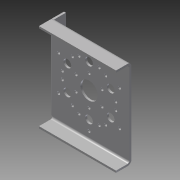
# Autodesk Inventor part: Plate 2 (Back)
Saved by Autodesk Inventor 2014 (Build 180170000, 170)
## iProperties
Created: 2014-01-12
Part Number: Plate 2 (Back)
Material: Steel
Document SubType Name: Sheet Metal
Designer: Andrew Toennies
Density: 7.85 g/cm^3
Sheet Metal Rule: Default
Appearance: Steel
Mass: 879.453 g
Surface Area: 760.069 cm^2
Volume: 112.032 cm^3
Author: Andrew Toennies
Autodesk Inventor part; units mm, degrees
ref_plane "YZ Plane" through (0, 0, 0) normal (1, 0, 0) x (0, 1, 0)
ref_plane "XZ Plane" through (0, 0, 0) normal (0, 1, 0) x (-1, 0, 0)
ref_plane "XY Plane" through (0, 0, 0) normal (0, 0, 1) x (1, 0, 0)
sketch "Sketch1" plane through (0, 0, 0) normal (0, 0, 1) x (1, 0, 0)
  circle A0 centre (0, 0) radius 66.675 construction
  circle A1 centre (0, 0) radius 14.2875
  circle A2 centre (0, 41.275) radius 6.3881
  line L0 (0, 0) -> (0, 41.275) construction
  circle A3 centre (0, 41.275) radius 16.637 construction
  circle A4 centre (0, 57.912) radius 2.3812
  circle A5 centre (16.637, 41.275) radius 2.3812
  circle A6 centre (0, 24.638) radius 2.3812
  circle A7 centre (-16.637, 41.275) radius 2.3813
  line L1 (0, 41.275) -> (0, 57.912) construction
  line L2 (-16.637, 41.275) -> (16.637, 41.275) construction
  circle A8 centre (-50.1533, 28.956) radius 2.3812
  circle A9 centre (-44.0637, 6.2294) radius 2.3813
  circle A10 centre (-35.7452, 20.6375) radius 6.3881
  circle A11 centre (-27.4267, 35.0456) radius 2.3812
  circle A12 centre (-21.3371, 12.319) radius 2.3812
  circle A13 centre (-50.1533, -28.956) radius 2.3812
  circle A14 centre (-27.4267, -35.0456) radius 2.3813
  circle A15 centre (-35.7452, -20.6375) radius 6.3881
  circle A16 centre (-44.0637, -6.2294) radius 2.3812
  circle A17 centre (-21.3371, -12.319) radius 2.3812
  circle A18 centre (0, -57.912) radius 2.3812
  circle A19 centre (16.637, -41.275) radius 2.3813
  circle A20 centre (0, -41.275) radius 6.3881
  circle A21 centre (-16.637, -41.275) radius 2.3812
  circle A22 centre (0, -24.638) radius 2.3812
  circle A23 centre (50.1533, -28.956) radius 2.3812
  circle A24 centre (44.0637, -6.2294) radius 2.3813
  circle A25 centre (35.7452, -20.6375) radius 6.3881
  circle A26 centre (27.4267, -35.0456) radius 2.3812
  circle A27 centre (21.3371, -12.319) radius 2.3812
  circle A28 centre (50.1533, 28.956) radius 2.3812
  circle A29 centre (27.4267, 35.0456) radius 2.3813
  circle A30 centre (35.7452, 20.6375) radius 6.3881
  circle A31 centre (44.0637, 6.2294) radius 2.3812
  circle A32 centre (21.3371, 12.319) radius 2.3812
  line L3 (-66.675, 66.675) -> (66.675, 66.675)
  line L4 (66.675, 66.675) -> (66.675, -66.675)
  line L5 (66.675, -66.675) -> (-66.675, -66.675)
  line L6 (-66.675, -66.675) -> (-66.675, 66.675)
  dimension "d2" = 133.35
  dimension "d3" = 28.575
  dimension "d4" = 12.7762
  dimension "d5" = 41.275
  dimension "d6" = 33.274
  dimension "d7" = 4.7625
  dimension "d8" = 4.7625
  dimension "d9" = 4.7625
  dimension "d10" = 4.7625
  dimension "d11" = 360
  measures "d2" diameter of A0
  measures "d3" diameter of A1
  measures "d4" diameter of A2
  measures "d5" distance of L0.start L0.end
  measures "d6" diameter of A3
  measures "d7" diameter of A4
  measures "d8" diameter of A5
  measures "d9" diameter of A6
  measures "d10" diameter of A7
extrude "Plate1" add sketch "Sketch1" along normal blind 3.175
sketch "Sketch3" plane through (66.675, -69.85, 6.35) normal (0, -1, 0) x (1, 0, 0)
  line L0 (-133.35, 0) -> (0, 0)
  line L1 (0, 0) -> (0, 69.85)
  line L2 (0, 69.85) -> (-133.35, 69.85)
  line L3 (-133.35, 69.85) -> (-133.35, 0)
  constraints: 6 end point, 1 horizontal, 1 perpendicular, 1 vertical
edge flange "Flange2" height 76.2 angle 90 thickness 3.175 bend radius 3.175 thickness toward (0, -1, 0) relief straight relief width 3.175 relief depth 1.5875 corner gap 3.175 corner form 0 edges at (0, -66.675, 3.175) (0, 66.675, 3.175) wall of the first edge with corners at (-66.675, -69.85, 6.35) (66.675, -69.85, 6.35) (66.675, -69.85, 76.2) (-66.675, -69.85, 76.2)
bend "Bend2"
corner "Corner2"
sketch "Sketch5" plane through (-66.675, 69.85, 76.2) normal (0, -1, 0) x (1, 0, 0)
  line L0 (38.7572, -36.5618) -> (41.6419, -43.3029) projected
  line L1 (41.6419, -43.3029) -> (48.9222, -44.1752) projected
  line L2 (48.9222, -44.1752) -> (53.3178, -38.3065) projected
  line L3 (53.3178, -38.3065) -> (50.4331, -31.5654) projected
  line L4 (50.4331, -31.5654) -> (43.1528, -30.6931) projected
  line L5 (43.1528, -30.6931) -> (38.7572, -36.5618) projected
  line L6 (53.3178, -38.3065) -> (38.7572, -36.5618) construction
  line L7 (48.9222, -44.1752) -> (43.1528, -30.6931) construction
  circle A0 centre (46.0375, -37.4342) radius 14.2875
  point P0 (66.675, -76.2)
  dimension "d39" = 28.575
  constraints: 4 end point, 2 midpoint, 2 parallel, 1 centre point
  measures "d39" diameter of A0
extrude "Cut2" cut sketch "Sketch5" against normal mid plane 2540 contours L5 L4 L3 L2 L1 L0 | A0
sketch "Sketch6" plane through (-66.675, 73.025, 76.2) normal (0, 1, 0) x (1, 0, 0)
  circle A0 centre (46.0375, 37.4342) radius 14.2875 projected
  line L0 (133.35, 69.85) -> (0, 69.85) projected
  line L1 (0, 0) -> (0, 69.85) projected
  line L2 (133.35, 0) -> (0, 0) projected
  line L3 (133.35, 69.85) -> (133.35, 0) projected
  arc A1 (20.7582, 24.1116) -> (62.3859, 13.9978) centre (46.0375, 37.4342) ccw
  line L4 (0, 63.5) -> (20.7582, 24.1116)
  line L5 (133.35, 63.5) -> (62.3859, 13.9978)
  point P0 (66.675, 76.2)
  dimension "d42" = 57.15
  dimension "d43" = 6.35
  dimension "d44" = 6.35
  constraints: 4 end point, 2 point on circle, 2 point on line, 2 tangent, 1 centre point, 1 coincident
  measures "d42" diameter of A1
  measures "d43" distance from line of L0 L4.start
  measures "d44" distance of L5.start L0.start
extrude "Cut3" cut sketch "Sketch6" against normal blind 254 contours L3 L2 L1 L4 A1 L5
fillet "Fillet1" radius 3.175 4 edges at (66.675, 71.4375, 12.7) (66.675, -71.4375, 12.7) (-66.675, 71.4375, 12.7) (-66.675, -71.4375, 12.7)
equation "\"d23\" = BendReliefWidth"
equation "\"d24\" = BendReliefDepth"
equation "\"d25\" = MinimumRemnant"
equation "\"d26\" = BendRadius"
equation "\"d30\" = CornerReliefSize"
equation "\"d31\" = GapSize"
equation "\"d32\" = JacobiRadiusSize"
equation "\"BendRadius\" = Thickness"
equation "\"BendReliefWidth\" = Thickness"
equation "\"BendReliefDepth\" = 0.5 * Thickness"
equation "\"CornerReliefSize\" = 4 * Thickness"
equation "\"MinimumRemnant\" = 2 * Thickness"
equation "\"TransitionRadius\" = BendRadius"
equation "\"JacobiRadiusSize\" = BendRadius"
equation "\"GapSize\" = Thickness"
equation "\"d12\" = BendRadius"
equation "\"Thickness\" = 3.175"
body "Solid1"
